Autodesk Inventor part; units mm, degrees
(part 3 of 6)
  line L1739 (82.2883, 113.1969) -> (82.3936, 113.3698)
  line L1740 (82.3936, 113.3698) -> (82.5145, 113.5317)
  line L1741 (82.5145, 113.5317) -> (82.6499, 113.6806)
  line L1742 (82.6499, 113.6806) -> (82.7991, 113.8163)
  line L1743 (82.7991, 113.8163) -> (82.9608, 113.9372)
  line L1744 (82.9608, 113.9372) -> (83.1339, 114.0423)
  line L1745 (83.1339, 114.0423) -> (83.3176, 114.1308)
  line L1746 (83.3176, 114.1308) -> (83.5105, 114.2015)
  line L1747 (83.5105, 114.2015) -> (83.7117, 114.2531)
  line L1748 (83.7117, 114.2531) -> (83.9201, 114.2848)
  line L1749 (83.9201, 114.2848) -> (84.1349, 114.2959)
  line L1750 (84.1349, 114.2959) -> (84.3495, 114.2848)
  line L1751 (84.3495, 114.2848) -> (84.5581, 114.2531)
  line L1752 (84.5581, 114.2531) -> (84.7593, 114.2015)
  line L1753 (84.7593, 114.2015) -> (84.9523, 114.1308)
  line L1754 (84.9523, 114.1308) -> (85.1359, 114.0423)
  line L1755 (85.1359, 114.0423) -> (85.309, 113.9372)
  line L1756 (85.309, 113.9372) -> (85.4708, 113.8163)
  line L1757 (85.4708, 113.8163) -> (85.6198, 113.6806)
  line L1758 (85.6198, 113.6806) -> (85.7553, 113.5317)
  line L1759 (85.7553, 113.5317) -> (85.8762, 113.3698)
  line L1760 (85.8762, 113.3698) -> (85.9815, 113.1969)
  line L1761 (85.9815, 113.1969) -> (86.0699, 113.0133)
  line L1762 (86.0699, 113.0133) -> (86.1405, 112.8203)
  line L1763 (86.1405, 112.8203) -> (86.1922, 112.6191)
  line L1764 (86.1922, 112.6191) -> (86.224, 112.4104)
  line L1765 (86.224, 112.4104) -> (86.2349, 112.1957)
  line L1766 (86.2349, 112.1957) -> (86.224, 111.9811)
  line L1767 (86.224, 111.9811) -> (86.1922, 111.7727)
  line L1768 (86.1922, 111.7727) -> (86.1405, 111.5711)
  line L1769 (86.1405, 111.5711) -> (86.0699, 111.3782)
  line L1770 (86.0699, 111.3782) -> (85.9815, 111.1949)
  line L1771 (85.9815, 111.1949) -> (85.8762, 111.0216)
  line L1772 (85.8762, 111.0216) -> (85.7553, 110.8601)
  line L1773 (85.7553, 110.8601) -> (85.6198, 110.7109)
  line L1774 (85.6198, 110.7109) -> (85.4708, 110.5752)
  line L1775 (85.4708, 110.5752) -> (85.309, 110.4546)
  line L1776 (85.309, 110.4546) -> (85.1359, 110.3492)
  line L1777 (85.1359, 110.3492) -> (84.9523, 110.261)
  line L1778 (84.9523, 110.261) -> (84.7593, 110.1903)
  line L1779 (84.7593, 110.1903) -> (84.5581, 110.1383)
  line L1780 (84.5581, 110.1383) -> (84.3495, 110.1066)
  line L1781 (84.3495, 110.1066) -> (84.1349, 110.0956)
  line L1782 (84.1349, 110.0956) -> (83.9201, 110.1066)
  line L1783 (83.9201, 110.1066) -> (83.7117, 110.1383)
  line L1784 (83.7117, 110.1383) -> (83.5105, 110.1903)
  line L1785 (83.5105, 110.1903) -> (83.3176, 110.261)
  line L1786 (83.3176, 110.261) -> (83.1339, 110.3492)
  line L1787 (83.1339, 110.3492) -> (82.9608, 110.4546)
  line L1788 (82.9608, 110.4546) -> (82.7991, 110.5752)
  line L1789 (82.7991, 110.5752) -> (82.6499, 110.7109)
  line L1790 (82.6499, 110.7109) -> (82.5145, 110.8601)
  line L1791 (82.5145, 110.8601) -> (82.3936, 111.0216)
  line L1792 (82.3936, 111.0216) -> (82.2883, 111.1949)
  line L1793 (82.2883, 111.1949) -> (82.2, 111.3782)
  line L1794 (82.2, 111.3782) -> (82.1294, 111.5711)
  line L1795 (82.1294, 111.5711) -> (82.0775, 111.7727)
  line L1796 (82.0775, 111.7727) -> (82.0458, 111.9811)
  line L1797 (82.0458, 111.9811) -> (82.035, 112.1957)
  line L1798 (12.0344, 112.1957) -> (12.0453, 112.4104)
  line L1799 (12.0453, 112.4104) -> (12.0771, 112.6191)
  line L1800 (12.0771, 112.6191) -> (12.1288, 112.8203)
  line L1801 (12.1288, 112.8203) -> (12.1994, 113.0133)
  line L1802 (12.1994, 113.0133) -> (12.288, 113.1969)
  line L1803 (12.288, 113.1969) -> (12.393, 113.3698)
  line L1804 (12.393, 113.3698) -> (12.514, 113.5317)
  line L1805 (12.514, 113.5317) -> (12.6495, 113.6806)
  line L1806 (12.6495, 113.6806) -> (12.7987, 113.8163)
  line L1807 (12.7987, 113.8163) -> (12.9603, 113.9372)
  line L1808 (12.9603, 113.9372) -> (13.1334, 114.0423)
  line L1809 (13.1334, 114.0423) -> (13.317, 114.1308)
  line L1810 (13.317, 114.1308) -> (13.5099, 114.2015)
  line L1811 (13.5099, 114.2015) -> (13.7111, 114.2531)
  line L1812 (13.7111, 114.2531) -> (13.9197, 114.2848)
  line L1813 (13.9197, 114.2848) -> (14.1344, 114.2959)
  line L1814 (14.1344, 114.2959) -> (14.3492, 114.2848)
  line L1815 (14.3492, 114.2848) -> (14.5576, 114.2531)
  line L1816 (14.5576, 114.2531) -> (14.759, 114.2015)
  line L1817 (14.759, 114.2015) -> (14.9519, 114.1308)
  line L1818 (14.9519, 114.1308) -> (15.1355, 114.0423)
  line L1819 (15.1355, 114.0423) -> (15.3086, 113.9372)
  line L1820 (15.3086, 113.9372) -> (15.4702, 113.8163)
  line L1821 (15.4702, 113.8163) -> (15.6194, 113.6806)
  line L1822 (15.6194, 113.6806) -> (15.7549, 113.5317)
  line L1823 (15.7549, 113.5317) -> (15.8759, 113.3698)
  line L1824 (15.8759, 113.3698) -> (15.9809, 113.1969)
  line L1825 (15.9809, 113.1969) -> (16.0695, 113.0133)
  line L1826 (16.0695, 113.0133) -> (16.1401, 112.8203)
  line L1827 (16.1401, 112.8203) -> (16.1918, 112.6191)
  line L1828 (16.1918, 112.6191) -> (16.2236, 112.4104)
  line L1829 (16.2236, 112.4104) -> (16.2345, 112.1957)
  line L1830 (16.2345, 112.1957) -> (16.2236, 111.9811)
  line L1831 (16.2236, 111.9811) -> (16.1918, 111.7727)
  line L1832 (16.1918, 111.7727) -> (16.1401, 111.5711)
  line L1833 (16.1401, 111.5711) -> (16.0695, 111.3782)
  line L1834 (16.0695, 111.3782) -> (15.9809, 111.1949)
  line L1835 (15.9809, 111.1949) -> (15.8759, 111.0216)
  line L1836 (15.8759, 111.0216) -> (15.7549, 110.8601)
  line L1837 (15.7549, 110.8601) -> (15.6194, 110.7109)
  line L1838 (15.6194, 110.7109) -> (15.4702, 110.5752)
  line L1839 (15.4702, 110.5752) -> (15.3086, 110.4546)
  line L1840 (15.3086, 110.4546) -> (15.1355, 110.3492)
  line L1841 (15.1355, 110.3492) -> (14.9519, 110.261)
  line L1842 (14.9519, 110.261) -> (14.759, 110.1903)
  line L1843 (14.759, 110.1903) -> (14.5576, 110.1383)
  line L1844 (14.5576, 110.1383) -> (14.3492, 110.1066)
  line L1845 (14.3492, 110.1066) -> (14.1344, 110.0956)
  line L1846 (14.1344, 110.0956) -> (13.9197, 110.1066)
  line L1847 (13.9197, 110.1066) -> (13.7111, 110.1383)
  line L1848 (13.7111, 110.1383) -> (13.5099, 110.1903)
  line L1849 (13.5099, 110.1903) -> (13.317, 110.261)
  line L1850 (13.317, 110.261) -> (13.1334, 110.3492)
  line L1851 (13.1334, 110.3492) -> (12.9603, 110.4546)
  line L1852 (12.9603, 110.4546) -> (12.7987, 110.5752)
  line L1853 (12.7987, 110.5752) -> (12.6495, 110.7109)
  line L1854 (12.6495, 110.7109) -> (12.514, 110.8601)
  line L1855 (12.514, 110.8601) -> (12.393, 111.0216)
  line L1856 (12.393, 111.0216) -> (12.288, 111.1949)
  line L1857 (12.288, 111.1949) -> (12.1994, 111.3782)
  line L1858 (12.1994, 111.3782) -> (12.1288, 111.5711)
  line L1859 (12.1288, 111.5711) -> (12.0771, 111.7727)
  line L1860 (12.0771, 111.7727) -> (12.0453, 111.9811)
  line L1861 (12.0453, 111.9811) -> (12.0344, 112.1957)
  line L1862 (26.0365, 112.1957) -> (26.0473, 112.4104)
  line L1863 (26.0473, 112.4104) -> (26.0792, 112.6191)
  line L1864 (26.0792, 112.6191) -> (26.1309, 112.8203)
  line L1865 (26.1309, 112.8203) -> (26.2015, 113.0133)
  line L1866 (26.2015, 113.0133) -> (26.2899, 113.1969)
  line L1867 (26.2899, 113.1969) -> (26.3951, 113.3698)
  line L1868 (26.3951, 113.3698) -> (26.516, 113.5317)
  line L1869 (26.516, 113.5317) -> (26.6516, 113.6806)
  line L1870 (26.6516, 113.6806) -> (26.8006, 113.8163)
  line L1871 (26.8006, 113.8163) -> (26.9624, 113.9372)
  line L1872 (26.9624, 113.9372) -> (27.1355, 114.0423)
  line L1873 (27.1355, 114.0423) -> (27.3191, 114.1308)
  line L1874 (27.3191, 114.1308) -> (27.512, 114.2015)
  line L1875 (27.512, 114.2015) -> (27.7132, 114.2531)
  line L1876 (27.7132, 114.2531) -> (27.9218, 114.2848)
  line L1877 (27.9218, 114.2848) -> (28.1364, 114.2959)
  line L1878 (28.1364, 114.2959) -> (28.3512, 114.2848)
  line L1879 (28.3512, 114.2848) -> (28.5597, 114.2531)
  line L1880 (28.5597, 114.2531) -> (28.7609, 114.2015)
  line L1881 (28.7609, 114.2015) -> (28.954, 114.1308)
  line L1882 (28.954, 114.1308) -> (29.1374, 114.0423)
  line L1883 (29.1374, 114.0423) -> (29.3105, 113.9372)
  line L1884 (29.3105, 113.9372) -> (29.4723, 113.8163)
  line L1885 (29.4723, 113.8163) -> (29.6214, 113.6806)
  line L1886 (29.6214, 113.6806) -> (29.7568, 113.5317)
  line L1887 (29.7568, 113.5317) -> (29.8778, 113.3698)
  line L1888 (29.8778, 113.3698) -> (29.983, 113.1969)
  line L1889 (29.983, 113.1969) -> (30.0714, 113.0133)
  line L1890 (30.0714, 113.0133) -> (30.142, 112.8203)
  line L1891 (30.142, 112.8203) -> (30.1939, 112.6191)
  line L1892 (30.1939, 112.6191) -> (30.2255, 112.4104)
  line L1893 (30.2255, 112.4104) -> (30.2364, 112.1957)
  line L1894 (30.2364, 112.1957) -> (30.2255, 111.9811)
  line L1895 (30.2255, 111.9811) -> (30.1939, 111.7727)
  line L1896 (30.1939, 111.7727) -> (30.142, 111.5711)
  line L1897 (30.142, 111.5711) -> (30.0714, 111.3782)
  line L1898 (30.0714, 111.3782) -> (29.983, 111.1949)
  line L1899 (29.983, 111.1949) -> (29.8778, 111.0216)
  line L1900 (29.8778, 111.0216) -> (29.7568, 110.8601)
  line L1901 (29.7568, 110.8601) -> (29.6214, 110.7109)
  line L1902 (29.6214, 110.7109) -> (29.4723, 110.5752)
  line L1903 (29.4723, 110.5752) -> (29.3105, 110.4546)
  line L1904 (29.3105, 110.4546) -> (29.1374, 110.3492)
  line L1905 (29.1374, 110.3492) -> (28.954, 110.261)
  line L1906 (28.954, 110.261) -> (28.7609, 110.1903)
  line L1907 (28.7609, 110.1903) -> (28.5597, 110.1383)
  line L1908 (28.5597, 110.1383) -> (28.3512, 110.1066)
  line L1909 (28.3512, 110.1066) -> (28.1364, 110.0956)
  line L1910 (28.1364, 110.0956) -> (27.9218, 110.1066)
  line L1911 (27.9218, 110.1066) -> (27.7132, 110.1383)
  line L1912 (27.7132, 110.1383) -> (27.512, 110.1903)
  line L1913 (27.512, 110.1903) -> (27.3191, 110.261)
  line L1914 (27.3191, 110.261) -> (27.1355, 110.3492)
  line L1915 (27.1355, 110.3492) -> (26.9624, 110.4546)
  line L1916 (26.9624, 110.4546) -> (26.8006, 110.5752)
  line L1917 (26.8006, 110.5752) -> (26.6516, 110.7109)
  line L1918 (26.6516, 110.7109) -> (26.516, 110.8601)
  line L1919 (26.516, 110.8601) -> (26.3951, 111.0216)
  line L1920 (26.3951, 111.0216) -> (26.2899, 111.1949)
  line L1921 (26.2899, 111.1949) -> (26.2015, 111.3782)
  line L1922 (26.2015, 111.3782) -> (26.1309, 111.5711)
  line L1923 (26.1309, 111.5711) -> (26.0792, 111.7727)
  line L1924 (26.0792, 111.7727) -> (26.0473, 111.9811)
  line L1925 (26.0473, 111.9811) -> (26.0365, 112.1957)
  line L1926 (40.0355, 112.1957) -> (40.0463, 112.4104)
  line L1927 (40.0463, 112.4104) -> (40.0782, 112.6191)
  line L1928 (40.0782, 112.6191) -> (40.1299, 112.8203)
  line L1929 (40.1299, 112.8203) -> (40.2005, 113.0133)
  line L1930 (40.2005, 113.0133) -> (40.289, 113.1969)
  line L1931 (40.289, 113.1969) -> (40.3941, 113.3698)
  line L1932 (40.3941, 113.3698) -> (40.515, 113.5317)
  line L1933 (40.515, 113.5317) -> (40.6506, 113.6806)
  line L1934 (40.6506, 113.6806) -> (40.7997, 113.8163)
  line L1935 (40.7997, 113.8163) -> (40.9613, 113.9372)
  line L1936 (40.9613, 113.9372) -> (41.1344, 114.0423)
  line L1937 (41.1344, 114.0423) -> (41.3181, 114.1308)
  line L1938 (41.3181, 114.1308) -> (41.511, 114.2015)
  line L1939 (41.511, 114.2015) -> (41.7122, 114.2531)
  line L1940 (41.7122, 114.2531) -> (41.9208, 114.2848)
  line L1941 (41.9208, 114.2848) -> (42.1354, 114.2959)
  line L1942 (42.1354, 114.2959) -> (42.3502, 114.2848)
  line L1943 (42.3502, 114.2848) -> (42.5586, 114.2531)
  line L1944 (42.5586, 114.2531) -> (42.76, 114.2015)
  line L1945 (42.76, 114.2015) -> (42.9529, 114.1308)
  line L1946 (42.9529, 114.1308) -> (43.1364, 114.0423)
  line L1947 (43.1364, 114.0423) -> (43.3097, 113.9372)
  line L1948 (43.3097, 113.9372) -> (43.4712, 113.8163)
  line L1949 (43.4712, 113.8163) -> (43.6204, 113.6806)
  line L1950 (43.6204, 113.6806) -> (43.756, 113.5317)
  line L1951 (43.756, 113.5317) -> (43.8769, 113.3698)
  line L1952 (43.8769, 113.3698) -> (43.982, 113.1969)
  line L1953 (43.982, 113.1969) -> (44.0705, 113.0133)
  line L1954 (44.0705, 113.0133) -> (44.1411, 112.8203)
  line L1955 (44.1411, 112.8203) -> (44.1928, 112.6191)
  line L1956 (44.1928, 112.6191) -> (44.2247, 112.4104)
  line L1957 (44.2247, 112.4104) -> (44.2355, 112.1957)
  line L1958 (44.2355, 112.1957) -> (44.2247, 111.9811)
  line L1959 (44.2247, 111.9811) -> (44.1928, 111.7727)
  line L1960 (44.1928, 111.7727) -> (44.1411, 111.5711)
  line L1961 (44.1411, 111.5711) -> (44.0705, 111.3782)
  line L1962 (44.0705, 111.3782) -> (43.982, 111.1949)
  line L1963 (43.982, 111.1949) -> (43.8769, 111.0216)
  line L1964 (43.8769, 111.0216) -> (43.756, 110.8601)
  line L1965 (43.756, 110.8601) -> (43.6204, 110.7109)
  line L1966 (43.6204, 110.7109) -> (43.4712, 110.5752)
  line L1967 (43.4712, 110.5752) -> (43.3097, 110.4546)
  line L1968 (43.3097, 110.4546) -> (43.1364, 110.3492)
  line L1969 (43.1364, 110.3492) -> (42.9529, 110.261)
  line L1970 (42.9529, 110.261) -> (42.76, 110.1903)
  line L1971 (42.76, 110.1903) -> (42.5586, 110.1383)
  line L1972 (42.5586, 110.1383) -> (42.3502, 110.1066)
  line L1973 (42.3502, 110.1066) -> (42.1354, 110.0956)
  line L1974 (42.1354, 110.0956) -> (41.9208, 110.1066)
  line L1975 (41.9208, 110.1066) -> (41.7122, 110.1383)
  line L1976 (41.7122, 110.1383) -> (41.511, 110.1903)
  line L1977 (41.511, 110.1903) -> (41.3181, 110.261)
  line L1978 (41.3181, 110.261) -> (41.1344, 110.3492)
  line L1979 (41.1344, 110.3492) -> (40.9613, 110.4546)
  line L1980 (40.9613, 110.4546) -> (40.7997, 110.5752)
  line L1981 (40.7997, 110.5752) -> (40.6506, 110.7109)
  line L1982 (40.6506, 110.7109) -> (40.515, 110.8601)
  line L1983 (40.515, 110.8601) -> (40.3941, 111.0216)
  line L1984 (40.3941, 111.0216) -> (40.289, 111.1949)
  line L1985 (40.289, 111.1949) -> (40.2005, 111.3782)
  line L1986 (40.2005, 111.3782) -> (40.1299, 111.5711)
  line L1987 (40.1299, 111.5711) -> (40.0782, 111.7727)
  line L1988 (40.0782, 111.7727) -> (40.0463, 111.9811)
  line L1989 (40.0463, 111.9811) -> (40.0355, 112.1957)
  line L1990 (54.0346, 112.1957) -> (54.0455, 112.4104)
  line L1991 (54.0455, 112.4104) -> (54.0773, 112.6191)
  line L1992 (54.0773, 112.6191) -> (54.1292, 112.8203)
  line L1993 (54.1292, 112.8203) -> (54.1996, 113.0133)
  line L1994 (54.1996, 113.0133) -> (54.2882, 113.1969)
  line L1995 (54.2882, 113.1969) -> (54.3934, 113.3698)
  line L1996 (54.3934, 113.3698) -> (54.5142, 113.5317)
  line L1997 (54.5142, 113.5317) -> (54.6497, 113.6806)
  line L1998 (54.6497, 113.6806) -> (54.7989, 113.8163)
  line L1999 (54.7989, 113.8163) -> (54.9605, 113.9372)
  line L2000 (54.9605, 113.9372) -> (55.1338, 114.0423)
  line L2001 (55.1338, 114.0423) -> (55.3172, 114.1308)
  line L2002 (55.3172, 114.1308) -> (55.5101, 114.2015)
  line L2003 (55.5101, 114.2015) -> (55.7115, 114.2531)
  line L2004 (55.7115, 114.2531) -> (55.9199, 114.2848)
  line L2005 (55.9199, 114.2848) -> (56.1347, 114.2959)
  line L2006 (56.1347, 114.2959) -> (56.3494, 114.2848)
  line L2007 (56.3494, 114.2848) -> (56.558, 114.2531)
  line L2008 (56.558, 114.2531) -> (56.7592, 114.2015)
  line L2009 (56.7592, 114.2015) -> (56.9521, 114.1308)
  line L2010 (56.9521, 114.1308) -> (57.1357, 114.0423)
  line L2011 (57.1357, 114.0423) -> (57.3088, 113.9372)
  line L2012 (57.3088, 113.9372) -> (57.4704, 113.8163)
  line L2013 (57.4704, 113.8163) -> (57.6196, 113.6806)
  line L2014 (57.6196, 113.6806) -> (57.7551, 113.5317)
  line L2015 (57.7551, 113.5317) -> (57.8761, 113.3698)
  line L2016 (57.8761, 113.3698) -> (57.9813, 113.1969)
  line L2017 (57.9813, 113.1969) -> (58.0697, 113.0133)
  line L2018 (58.0697, 113.0133) -> (58.1403, 112.8203)
  line L2019 (58.1403, 112.8203) -> (58.192, 112.6191)
  line L2020 (58.192, 112.6191) -> (58.2238, 112.4104)
  line L2021 (58.2238, 112.4104) -> (58.2347, 112.1957)
  line L2022 (58.2347, 112.1957) -> (58.2238, 111.9811)
  line L2023 (58.2238, 111.9811) -> (58.192, 111.7727)
  line L2024 (58.192, 111.7727) -> (58.1403, 111.5711)
  line L2025 (58.1403, 111.5711) -> (58.0697, 111.3782)
  line L2026 (58.0697, 111.3782) -> (57.9813, 111.1949)
  line L2027 (57.9813, 111.1949) -> (57.8761, 111.0216)
  line L2028 (57.8761, 111.0216) -> (57.7551, 110.8601)
  line L2029 (57.7551, 110.8601) -> (57.6196, 110.7109)
  line L2030 (57.6196, 110.7109) -> (57.4704, 110.5752)
  line L2031 (57.4704, 110.5752) -> (57.3088, 110.4546)
  line L2032 (57.3088, 110.4546) -> (57.1357, 110.3492)
  line L2033 (57.1357, 110.3492) -> (56.9521, 110.261)
  line L2034 (56.9521, 110.261) -> (56.7592, 110.1903)
  line L2035 (56.7592, 110.1903) -> (56.558, 110.1383)
  line L2036 (56.558, 110.1383) -> (56.3494, 110.1066)
  line L2037 (56.3494, 110.1066) -> (56.1347, 110.0956)
  line L2038 (56.1347, 110.0956) -> (55.9199, 110.1066)
  line L2039 (55.9199, 110.1066) -> (55.7115, 110.1383)
  line L2040 (55.7115, 110.1383) -> (55.5101, 110.1903)
  line L2041 (55.5101, 110.1903) -> (55.3172, 110.261)
  line L2042 (55.3172, 110.261) -> (55.1338, 110.3492)
  line L2043 (55.1338, 110.3492) -> (54.9605, 110.4546)
  line L2044 (54.9605, 110.4546) -> (54.7989, 110.5752)
  line L2045 (54.7989, 110.5752) -> (54.6497, 110.7109)
  line L2046 (54.6497, 110.7109) -> (54.5142, 110.8601)
  line L2047 (54.5142, 110.8601) -> (54.3934, 111.0216)
  line L2048 (54.3934, 111.0216) -> (54.2882, 111.1949)
  line L2049 (54.2882, 111.1949) -> (54.1996, 111.3782)
  line L2050 (54.1996, 111.3782) -> (54.1292, 111.5711)
  line L2051 (54.1292, 111.5711) -> (54.0773, 111.7727)
  line L2052 (54.0773, 111.7727) -> (54.0455, 111.9811)
  line L2053 (54.0455, 111.9811) -> (54.0346, 112.1957)
  line L2054 (96.0253, 112.1957) -> (96.0362, 112.4104)
  line L2055 (96.0362, 112.4104) -> (96.0679, 112.6191)
  line L2056 (96.0679, 112.6191) -> (96.1197, 112.8203)
  line L2057 (96.1197, 112.8203) -> (96.1903, 113.0133)
  line L2058 (96.1903, 113.0133) -> (96.2787, 113.1969)
  line L2059 (96.2787, 113.1969) -> (96.384, 113.3698)
  line L2060 (96.384, 113.3698) -> (96.5049, 113.5317)
  line L2061 (96.5049, 113.5317) -> (96.6403, 113.6806)
  line L2062 (96.6403, 113.6806) -> (96.7894, 113.8163)
  line L2063 (96.7894, 113.8163) -> (96.9512, 113.9372)
  line L2064 (96.9512, 113.9372) -> (97.1243, 114.0423)
  line L2065 (97.1243, 114.0423) -> (97.3079, 114.1308)
  line L2066 (97.3079, 114.1308) -> (97.5009, 114.2015)
  line L2067 (97.5009, 114.2015) -> (97.702, 114.2531)
  line L2068 (97.702, 114.2531) -> (97.9105, 114.2848)
  line L2069 (97.9105, 114.2848) -> (98.1253, 114.2959)
  line L2070 (98.1253, 114.2959) -> (98.3399, 114.2848)
  line L2071 (98.3399, 114.2848) -> (98.5485, 114.2531)
  line L2072 (98.5485, 114.2531) -> (98.7497, 114.2015)
  line L2073 (98.7497, 114.2015) -> (98.9426, 114.1308)
  line L2074 (98.9426, 114.1308) -> (99.1262, 114.0423)
  line L2075 (99.1262, 114.0423) -> (99.2994, 113.9372)
  line L2076 (99.2994, 113.9372) -> (99.4611, 113.8163)
  line L2077 (99.4611, 113.8163) -> (99.6101, 113.6806)
  line L2078 (99.6101, 113.6806) -> (99.7457, 113.5317)
  line L2079 (99.7457, 113.5317) -> (99.8666, 113.3698)
  line L2080 (99.8666, 113.3698) -> (99.9718, 113.1969)
  line L2081 (99.9718, 113.1969) -> (100.0602, 113.0133)
  line L2082 (100.0602, 113.0133) -> (100.1308, 112.8203)
  line L2083 (100.1308, 112.8203) -> (100.1827, 112.6191)
  line L2084 (100.1827, 112.6191) -> (100.2144, 112.4104)
  line L2085 (100.2144, 112.4104) -> (100.2252, 112.1957)
  line L2086 (100.2252, 112.1957) -> (100.2144, 111.9811)
  line L2087 (100.2144, 111.9811) -> (100.1827, 111.7727)
  line L2088 (100.1827, 111.7727) -> (100.1308, 111.5711)
  line L2089 (100.1308, 111.5711) -> (100.0602, 111.3782)
  line L2090 (100.0602, 111.3782) -> (99.9718, 111.1949)
  line L2091 (99.9718, 111.1949) -> (99.8666, 111.0216)
  line L2092 (99.8666, 111.0216) -> (99.7457, 110.8601)
  line L2093 (99.7457, 110.8601) -> (99.6101, 110.7109)
  line L2094 (99.6101, 110.7109) -> (99.4611, 110.5752)
  line L2095 (99.4611, 110.5752) -> (99.2994, 110.4546)
  line L2096 (99.2994, 110.4546) -> (99.1262, 110.3492)
  line L2097 (99.1262, 110.3492) -> (98.9426, 110.261)
  line L2098 (98.9426, 110.261) -> (98.7497, 110.1903)
  line L2099 (98.7497, 110.1903) -> (98.5485, 110.1383)
  line L2100 (98.5485, 110.1383) -> (98.3399, 110.1066)
  line L2101 (98.3399, 110.1066) -> (98.1253, 110.0956)
  line L2102 (98.1253, 110.0956) -> (97.9105, 110.1066)
  line L2103 (97.9105, 110.1066) -> (97.702, 110.1383)
  line L2104 (97.702, 110.1383) -> (97.5009, 110.1903)
  line L2105 (97.5009, 110.1903) -> (97.3079, 110.261)
  line L2106 (97.3079, 110.261) -> (97.1243, 110.3492)
  line L2107 (97.1243, 110.3492) -> (96.9512, 110.4546)
  line L2108 (96.9512, 110.4546) -> (96.7894, 110.5752)
  line L2109 (96.7894, 110.5752) -> (96.6403, 110.7109)
  line L2110 (96.6403, 110.7109) -> (96.5049, 110.8601)
  line L2111 (96.5049, 110.8601) -> (96.384, 111.0216)
  line L2112 (96.384, 111.0216) -> (96.2787, 111.1949)
  line L2113 (96.2787, 111.1949) -> (96.1903, 111.3782)
  line L2114 (96.1903, 111.3782) -> (96.1197, 111.5711)
  line L2115 (96.1197, 111.5711) -> (96.0679, 111.7727)
  line L2116 (96.0679, 111.7727) -> (96.0362, 111.9811)
  line L2117 (96.0362, 111.9811) -> (96.0253, 112.1957)
  line L2118 (110.0253, 112.1957) -> (110.0363, 112.4104)
  line L2119 (110.0363, 112.4104) -> (110.068, 112.6191)
  line L2120 (110.068, 112.6191) -> (110.1197, 112.8203)
  line L2121 (110.1197, 112.8203) -> (110.1903, 113.0133)
  line L2122 (110.1903, 113.0133) -> (110.2789, 113.1969)
  line L2123 (110.2789, 113.1969) -> (110.384, 113.3698)
  line L2124 (110.384, 113.3698) -> (110.5049, 113.5317)
  line L2125 (110.5049, 113.5317) -> (110.6406, 113.6806)
  line L2126 (110.6406, 113.6806) -> (110.7898, 113.8163)
  line L2127 (110.7898, 113.8163) -> (110.9514, 113.9372)
  line L2128 (110.9514, 113.9372) -> (111.1243, 114.0423)
  line L2129 (111.1243, 114.0423) -> (111.3079, 114.1308)
  line L2130 (111.3079, 114.1308) -> (111.5009, 114.2015)
  line L2131 (111.5009, 114.2015) -> (111.7024, 114.2531)
  line L2132 (111.7024, 114.2531) -> (111.9108, 114.2848)
  line L2133 (111.9108, 114.2848) -> (112.1255, 114.2959)
  line L2134 (112.1255, 114.2959) -> (112.3401, 114.2848)
  line L2135 (112.3401, 114.2848) -> (112.5489, 114.2531)
  line L2136 (112.5489, 114.2531) -> (112.7501, 114.2015)
  line L2137 (112.7501, 114.2015) -> (112.943, 114.1308)
  line L2138 (112.943, 114.1308) -> (113.1266, 114.0423)
  line L2139 (113.1266, 114.0423) -> (113.2995, 113.9372)
  line L2140 (113.2995, 113.9372) -> (113.4611, 113.8163)
  line L2141 (113.4611, 113.8163) -> (113.6103, 113.6806)
  line L2142 (113.6103, 113.6806) -> (113.746, 113.5317)
  line L2143 (113.746, 113.5317) -> (113.867, 113.3698)
  line L2144 (113.867, 113.3698) -> (113.972, 113.1969)
  line L2145 (113.972, 113.1969) -> (114.0606, 113.0133)
  line L2146 (114.0606, 113.0133) -> (114.1312, 112.8203)
  line L2147 (114.1312, 112.8203) -> (114.1829, 112.6191)
  line L2148 (114.1829, 112.6191) -> (114.2146, 112.4104)
  line L2149 (114.2146, 112.4104) -> (114.2256, 112.1957)
  line L2150 (114.2256, 112.1957) -> (114.2146, 111.9811)
  line L2151 (114.2146, 111.9811) -> (114.1829, 111.7727)
  line L2152 (114.1829, 111.7727) -> (114.1312, 111.5711)
  line L2153 (114.1312, 111.5711) -> (114.0606, 111.3782)
  line L2154 (114.0606, 111.3782) -> (113.972, 111.1949)
  line L2155 (113.972, 111.1949) -> (113.867, 111.0216)
  line L2156 (113.867, 111.0216) -> (113.746, 110.8601)
  line L2157 (113.746, 110.8601) -> (113.6103, 110.7109)
  line L2158 (113.6103, 110.7109) -> (113.4611, 110.5752)
  line L2159 (113.4611, 110.5752) -> (113.2995, 110.4546)
  line L2160 (113.2995, 110.4546) -> (113.1266, 110.3492)
  line L2161 (113.1266, 110.3492) -> (112.943, 110.261)
  line L2162 (112.943, 110.261) -> (112.7501, 110.1903)
  line L2163 (112.7501, 110.1903) -> (112.5489, 110.1383)
  line L2164 (112.5489, 110.1383) -> (112.3401, 110.1066)
  line L2165 (112.3401, 110.1066) -> (112.1255, 110.0956)
  line L2166 (112.1255, 110.0956) -> (111.9108, 110.1066)
  line L2167 (111.9108, 110.1066) -> (111.7024, 110.1383)
  line L2168 (111.7024, 110.1383) -> (111.5009, 110.1903)
  line L2169 (111.5009, 110.1903) -> (111.3079, 110.261)
  line L2170 (111.3079, 110.261) -> (111.1243, 110.3492)
  line L2171 (111.1243, 110.3492) -> (110.9514, 110.4546)
  line L2172 (110.9514, 110.4546) -> (110.7898, 110.5752)
  line L2173 (110.7898, 110.5752) -> (110.6406, 110.7109)
  line L2174 (110.6406, 110.7109) -> (110.5049, 110.8601)
  line L2175 (110.5049, 110.8601) -> (110.384, 111.0216)
  line L2176 (110.384, 111.0216) -> (110.2789, 111.1949)
  line L2177 (110.2789, 111.1949) -> (110.1903, 111.3782)
  line L2178 (110.1903, 111.3782) -> (110.1197, 111.5711)
  line L2179 (110.1197, 111.5711) -> (110.068, 111.7727)
  line L2180 (110.068, 111.7727) -> (110.0363, 111.9811)
  line L2181 (110.0363, 111.9811) -> (110.0253, 112.1957)
  line L2182 (54.0346, 185.1932) -> (54.0455, 185.408)
  line L2183 (54.0455, 185.408) -> (54.0773, 185.6164)
  line L2184 (54.0773, 185.6164) -> (54.1292, 185.8178)
  line L2185 (54.1292, 185.8178) -> (54.1996, 186.0107)
  line L2186 (54.1996, 186.0107) -> (54.2882, 186.1941)
  line L2187 (54.2882, 186.1941) -> (54.3934, 186.3673)
  line L2188 (54.3934, 186.3673) -> (54.5142, 186.529)
  line L2189 (54.5142, 186.529) -> (54.6497, 186.6782)
  line L2190 (54.6497, 186.6782) -> (54.7989, 186.8137)
  line L2191 (54.7989, 186.8137) -> (54.9605, 186.9345)
  line L2192 (54.9605, 186.9345) -> (55.1338, 187.0397)
  line L2193 (55.1338, 187.0397) -> (55.3172, 187.1281)
  line L2194 (55.3172, 187.1281) -> (55.5101, 187.1987)
  line L2195 (55.5101, 187.1987) -> (55.7115, 187.2506)
  line L2196 (55.7115, 187.2506) -> (55.9199, 187.2823)
  line L2197 (55.9199, 187.2823) -> (56.1347, 187.2931)
  line L2198 (56.1347, 187.2931) -> (56.3494, 187.2823)
  line L2199 (56.3494, 187.2823) -> (56.558, 187.2506)
  line L2200 (56.558, 187.2506) -> (56.7592, 187.1987)
  line L2201 (56.7592, 187.1987) -> (56.9521, 187.1281)
  line L2202 (56.9521, 187.1281) -> (57.1357, 187.0397)
  line L2203 (57.1357, 187.0397) -> (57.3088, 186.9345)
  line L2204 (57.3088, 186.9345) -> (57.4704, 186.8137)
  line L2205 (57.4704, 186.8137) -> (57.6196, 186.6782)
  line L2206 (57.6196, 186.6782) -> (57.7551, 186.529)
  line L2207 (57.7551, 186.529) -> (57.8761, 186.3673)
  line L2208 (57.8761, 186.3673) -> (57.9813, 186.1941)
  line L2209 (57.9813, 186.1941) -> (58.0697, 186.0107)
  line L2210 (58.0697, 186.0107) -> (58.1403, 185.8178)
  line L2211 (58.1403, 185.8178) -> (58.192, 185.6164)
  line L2212 (58.192, 185.6164) -> (58.2238, 185.408)
  line L2213 (58.2238, 185.408) -> (58.2347, 185.1932)
  line L2214 (58.2347, 185.1932) -> (58.2238, 184.9785)
  line L2215 (58.2238, 184.9785) -> (58.192, 184.7699)
  line L2216 (58.192, 184.7699) -> (58.1403, 184.5688)
  line L2217 (58.1403, 184.5688) -> (58.0697, 184.3758)
  line L2218 (58.0697, 184.3758) -> (57.9813, 184.1922)
  line L2219 (57.9813, 184.1922) -> (57.8761, 184.0191)
  line L2220 (57.8761, 184.0191) -> (57.7551, 183.8573)
  line L2221 (57.7551, 183.8573) -> (57.6196, 183.7083)
  line L2222 (57.6196, 183.7083) -> (57.4704, 183.5728)
  line L2223 (57.4704, 183.5728) -> (57.3088, 183.4519)
  line L2224 (57.3088, 183.4519) -> (57.1357, 183.3466)
  line L2225 (57.1357, 183.3466) -> (56.9521, 183.2582)
  line L2226 (56.9521, 183.2582) -> (56.7592, 183.1876)
  line L2227 (56.7592, 183.1876) -> (56.558, 183.1359)
  line L2228 (56.558, 183.1359) -> (56.3494, 183.1041)
  line L2229 (56.3494, 183.1041) -> (56.1347, 183.0932)
  line L2230 (56.1347, 183.0932) -> (55.9199, 183.1041)
  line L2231 (55.9199, 183.1041) -> (55.7115, 183.1359)
  line L2232 (55.7115, 183.1359) -> (55.5101, 183.1876)
  line L2233 (55.5101, 183.1876) -> (55.3172, 183.2582)
  line L2234 (55.3172, 183.2582) -> (55.1338, 183.3466)
  line L2235 (55.1338, 183.3466) -> (54.9605, 183.4519)
  line L2236 (54.9605, 183.4519) -> (54.7989, 183.5728)
  line L2237 (54.7989, 183.5728) -> (54.6497, 183.7083)
  line L2238 (54.6497, 183.7083) -> (54.5142, 183.8573)
  line L2239 (54.5142, 183.8573) -> (54.3934, 184.0191)
  line L2240 (54.3934, 184.0191) -> (54.2882, 184.1922)
  line L2241 (54.2882, 184.1922) -> (54.1996, 184.3758)
  line L2242 (54.1996, 184.3758) -> (54.1292, 184.5688)
  line L2243 (54.1292, 184.5688) -> (54.0773, 184.7699)
  line L2244 (54.0773, 184.7699) -> (54.0455, 184.9785)
  line L2245 (54.0455, 184.9785) -> (54.0346, 185.1932)
  line L2246 (82.035, 185.1932) -> (82.0458, 185.408)
  line L2247 (82.0458, 185.408) -> (82.0775, 185.6164)
  line L2248 (82.0775, 185.6164) -> (82.1294, 185.8178)
  line L2249 (82.1294, 185.8178) -> (82.2, 186.0107)
  line L2250 (82.2, 186.0107) -> (82.2883, 186.1941)
  line L2251 (82.2883, 186.1941) -> (82.3936, 186.3673)
  line L2252 (82.3936, 186.3673) -> (82.5145, 186.529)
  line L2253 (82.5145, 186.529) -> (82.6499, 186.6782)
  line L2254 (82.6499, 186.6782) -> (82.7991, 186.8137)
  line L2255 (82.7991, 186.8137) -> (82.9608, 186.9345)
  line L2256 (82.9608, 186.9345) -> (83.1339, 187.0397)
  line L2257 (83.1339, 187.0397) -> (83.3176, 187.1281)
  line L2258 (83.3176, 187.1281) -> (83.5105, 187.1987)
  line L2259 (83.5105, 187.1987) -> (83.7117, 187.2506)
  line L2260 (83.7117, 187.2506) -> (83.9201, 187.2823)
  line L2261 (83.9201, 187.2823) -> (84.1349, 187.2931)
  line L2262 (84.1349, 187.2931) -> (84.3495, 187.2823)
  line L2263 (84.3495, 187.2823) -> (84.5581, 187.2506)
  line L2264 (84.5581, 187.2506) -> (84.7593, 187.1987)
  line L2265 (84.7593, 187.1987) -> (84.9523, 187.1281)
  line L2266 (84.9523, 187.1281) -> (85.1359, 187.0397)
  line L2267 (85.1359, 187.0397) -> (85.309, 186.9345)
  line L2268 (85.309, 186.9345) -> (85.4708, 186.8137)
  line L2269 (85.4708, 186.8137) -> (85.6198, 186.6782)
  line L2270 (85.6198, 186.6782) -> (85.7553, 186.529)
  line L2271 (85.7553, 186.529) -> (85.8762, 186.3673)
  line L2272 (85.8762, 186.3673) -> (85.9815, 186.1941)
  line L2273 (85.9815, 186.1941) -> (86.0699, 186.0107)
  line L2274 (86.0699, 186.0107) -> (86.1405, 185.8178)
  line L2275 (86.1405, 185.8178) -> (86.1922, 185.6164)
  line L2276 (86.1922, 185.6164) -> (86.224, 185.408)
  line L2277 (86.224, 185.408) -> (86.2349, 185.1932)
  line L2278 (86.2349, 185.1932) -> (86.224, 184.9785)
  line L2279 (86.224, 184.9785) -> (86.1922, 184.7699)
  line L2280 (86.1922, 184.7699) -> (86.1405, 184.5688)
  line L2281 (86.1405, 184.5688) -> (86.0699, 184.3758)
  line L2282 (86.0699, 184.3758) -> (85.9815, 184.1922)
  line L2283 (85.9815, 184.1922) -> (85.8762, 184.0191)
  line L2284 (85.8762, 184.0191) -> (85.7553, 183.8573)
  line L2285 (85.7553, 183.8573) -> (85.6198, 183.7083)
  line L2286 (85.6198, 183.7083) -> (85.4708, 183.5728)
  line L2287 (85.4708, 183.5728) -> (85.309, 183.4519)
  line L2288 (85.309, 183.4519) -> (85.1359, 183.3466)
  line L2289 (85.1359, 183.3466) -> (84.9523, 183.2582)
  line L2290 (84.9523, 183.2582) -> (84.7593, 183.1876)
  line L2291 (84.7593, 183.1876) -> (84.5581, 183.1359)
  line L2292 (84.5581, 183.1359) -> (84.3495, 183.1041)
  line L2293 (84.3495, 183.1041) -> (84.1349, 183.0932)
  line L2294 (84.1349, 183.0932) -> (83.9201, 183.1041)
  line L2295 (83.9201, 183.1041) -> (83.7117, 183.1359)
  line L2296 (83.7117, 183.1359) -> (83.5105, 183.1876)
  line L2297 (83.5105, 183.1876) -> (83.3176, 183.2582)
  line L2298 (83.3176, 183.2582) -> (83.1339, 183.3466)
  line L2299 (83.1339, 183.3466) -> (82.9608, 183.4519)
  line L2300 (82.9608, 183.4519) -> (82.7991, 183.5728)
  line L2301 (82.7991, 183.5728) -> (82.6499, 183.7083)
  line L2302 (82.6499, 183.7083) -> (82.5145, 183.8573)
  line L2303 (82.5145, 183.8573) -> (82.3936, 184.0191)
  line L2304 (82.3936, 184.0191) -> (82.2883, 184.1922)
  line L2305 (82.2883, 184.1922) -> (82.2, 184.3758)
  line L2306 (82.2, 184.3758) -> (82.1294, 184.5688)
  line L2307 (82.1294, 184.5688) -> (82.0775, 184.7699)
  line L2308 (82.0775, 184.7699) -> (82.0458, 184.9785)
  line L2309 (82.0458, 184.9785) -> (82.035, 185.1932)
  line L2310 (68.0346, 185.1932) -> (68.0455, 185.408)
  line L2311 (68.0455, 185.408) -> (68.0772, 185.6164)
  line L2312 (68.0772, 185.6164) -> (68.129, 185.8178)
  line L2313 (68.129, 185.8178) -> (68.1996, 186.0107)
  line L2314 (68.1996, 186.0107) -> (68.288, 186.1941)
  line L2315 (68.288, 186.1941) -> (68.3932, 186.3673)
  line L2316 (68.3932, 186.3673) -> (68.5142, 186.529)
  line L2317 (68.5142, 186.529) -> (68.6496, 186.6782)
  line L2318 (68.6496, 186.6782) -> (68.7987, 186.8137)
  line L2319 (68.7987, 186.8137) -> (68.9605, 186.9345)
  line L2320 (68.9605, 186.9345) -> (69.1336, 187.0397)
  line L2321 (69.1336, 187.0397) -> (69.317, 187.1281)
  line L2322 (69.317, 187.1281) -> (69.5101, 187.1987)
  line L2323 (69.5101, 187.1987) -> (69.7113, 187.2506)
  line L2324 (69.7113, 187.2506) -> (69.9198, 187.2823)
  line L2325 (69.9198, 187.2823) -> (70.1346, 187.2931)
  line L2326 (70.1346, 187.2931) -> (70.3492, 187.2823)
  line L2327 (70.3492, 187.2823) -> (70.5578, 187.2506)
  line L2328 (70.5578, 187.2506) -> (70.759, 187.1987)
  line L2329 (70.759, 187.1987) -> (70.9519, 187.1281)
  line L2330 (70.9519, 187.1281) -> (71.1355, 187.0397)
  line L2331 (71.1355, 187.0397) -> (71.3087, 186.9345)
  line L2332 (71.3087, 186.9345) -> (71.4704, 186.8137)
  line L2333 (71.4704, 186.8137) -> (71.6194, 186.6782)
  line L2334 (71.6194, 186.6782) -> (71.755, 186.529)
  line L2335 (71.755, 186.529) -> (71.8759, 186.3673)
  line L2336 (71.8759, 186.3673) -> (71.9811, 186.1941)
  line L2337 (71.9811, 186.1941) -> (72.0695, 186.0107)
  line L2338 (72.0695, 186.0107) -> (72.1401, 185.8178)
  line L2339 (72.1401, 185.8178) -> (72.1918, 185.6164)
  line L2340 (72.1918, 185.6164) -> (72.2237, 185.408)
  line L2341 (72.2237, 185.408) -> (72.2345, 185.1932)
  line L2342 (72.2345, 185.1932) -> (72.2237, 184.9785)
  line L2343 (72.2237, 184.9785) -> (72.1918, 184.7699)
  line L2344 (72.1918, 184.7699) -> (72.1401, 184.5688)
  line L2345 (72.1401, 184.5688) -> (72.0695, 184.3758)
  line L2346 (72.0695, 184.3758) -> (71.9811, 184.1922)
  line L2347 (71.9811, 184.1922) -> (71.8759, 184.0191)
  line L2348 (71.8759, 184.0191) -> (71.755, 183.8573)
  line L2349 (71.755, 183.8573) -> (71.6194, 183.7083)
  line L2350 (71.6194, 183.7083) -> (71.4704, 183.5728)
  line L2351 (71.4704, 183.5728) -> (71.3087, 183.4519)
  line L2352 (71.3087, 183.4519) -> (71.1355, 183.3466)
  line L2353 (71.1355, 183.3466) -> (70.9519, 183.2582)
  line L2354 (70.9519, 183.2582) -> (70.759, 183.1876)
  line L2355 (70.759, 183.1876) -> (70.5578, 183.1359)
  line L2356 (70.5578, 183.1359) -> (70.3492, 183.1041)
  line L2357 (70.3492, 183.1041) -> (70.1346, 183.0932)
  line L2358 (70.1346, 183.0932) -> (69.9198, 183.1041)
  line L2359 (69.9198, 183.1041) -> (69.7113, 183.1359)
  line L2360 (69.7113, 183.1359) -> (69.5101, 183.1876)
  line L2361 (69.5101, 183.1876) -> (69.317, 183.2582)
  line L2362 (69.317, 183.2582) -> (69.1336, 183.3466)
  line L2363 (69.1336, 183.3466) -> (68.9605, 183.4519)
  line L2364 (68.9605, 183.4519) -> (68.7987, 183.5728)
  line L2365 (68.7987, 183.5728) -> (68.6496, 183.7083)
  line L2366 (68.6496, 183.7083) -> (68.5142, 183.8573)
  line L2367 (68.5142, 183.8573) -> (68.3932, 184.0191)
  line L2368 (68.3932, 184.0191) -> (68.288, 184.1922)
  line L2369 (68.288, 184.1922) -> (68.1996, 184.3758)
  line L2370 (68.1996, 184.3758) -> (68.129, 184.5688)
  line L2371 (68.129, 184.5688) -> (68.0772, 184.7699)
  line L2372 (68.0772, 184.7699) -> (68.0455, 184.9785)
  line L2373 (68.0455, 184.9785) -> (68.0346, 185.1932)
  line L2374 (96.0253, 185.1932) -> (96.0362, 185.408)
  line L2375 (96.0362, 185.408) -> (96.0679, 185.6164)
  line L2376 (96.0679, 185.6164) -> (96.1197, 185.8178)
  line L2377 (96.1197, 185.8178) -> (96.1903, 186.0107)
  line L2378 (96.1903, 186.0107) -> (96.2787, 186.1941)
  line L2379 (96.2787, 186.1941) -> (96.384, 186.3673)
  line L2380 (96.384, 186.3673) -> (96.5049, 186.529)
  line L2381 (96.5049, 186.529) -> (96.6403, 186.6782)
  line L2382 (96.6403, 186.6782) -> (96.7894, 186.8137)
  line L2383 (96.7894, 186.8137) -> (96.9512, 186.9345)
  line L2384 (96.9512, 186.9345) -> (97.1243, 187.0397)
  line L2385 (97.1243, 187.0397) -> (97.3079, 187.1281)
  line L2386 (97.3079, 187.1281) -> (97.5009, 187.1987)
  line L2387 (97.5009, 187.1987) -> (97.702, 187.2506)
  line L2388 (97.702, 187.2506) -> (97.9105, 187.2823)
  line L2389 (97.9105, 187.2823) -> (98.1253, 187.2931)
  line L2390 (98.1253, 187.2931) -> (98.3399, 187.2823)
  line L2391 (98.3399, 187.2823) -> (98.5485, 187.2506)
  line L2392 (98.5485, 187.2506) -> (98.7497, 187.1987)
  line L2393 (98.7497, 187.1987) -> (98.9426, 187.1281)
  line L2394 (98.9426, 187.1281) -> (99.1262, 187.0397)
  line L2395 (99.1262, 187.0397) -> (99.2994, 186.9345)
  line L2396 (99.2994, 186.9345) -> (99.4611, 186.8137)
  line L2397 (99.4611, 186.8137) -> (99.6101, 186.6782)
  line L2398 (99.6101, 186.6782) -> (99.7457, 186.529)
  line L2399 (99.7457, 186.529) -> (99.8666, 186.3673)
  line L2400 (99.8666, 186.3673) -> (99.9718, 186.1941)
  line L2401 (99.9718, 186.1941) -> (100.0602, 186.0107)
  line L2402 (100.0602, 186.0107) -> (100.1308, 185.8178)
  line L2403 (100.1308, 185.8178) -> (100.1827, 185.6164)
  line L2404 (100.1827, 185.6164) -> (100.2144, 185.408)
  line L2405 (100.2144, 185.408) -> (100.2252, 185.1932)
  line L2406 (100.2252, 185.1932) -> (100.2144, 184.9785)
  line L2407 (100.2144, 184.9785) -> (100.1827, 184.7699)
  line L2408 (100.1827, 184.7699) -> (100.1308, 184.5688)
  line L2409 (100.1308, 184.5688) -> (100.0602, 184.3758)
  line L2410 (100.0602, 184.3758) -> (99.9718, 184.1922)
  line L2411 (99.9718, 184.1922) -> (99.8666, 184.0191)
  line L2412 (99.8666, 184.0191) -> (99.7457, 183.8573)
  line L2413 (99.7457, 183.8573) -> (99.6101, 183.7083)
  line L2414 (99.6101, 183.7083) -> (99.4611, 183.5728)
  line L2415 (99.4611, 183.5728) -> (99.2994, 183.4519)
  line L2416 (99.2994, 183.4519) -> (99.1262, 183.3466)
  line L2417 (99.1262, 183.3466) -> (98.9426, 183.2582)
  line L2418 (98.9426, 183.2582) -> (98.7497, 183.1876)
  line L2419 (98.7497, 183.1876) -> (98.5485, 183.1359)
  line L2420 (98.5485, 183.1359) -> (98.3399, 183.1041)
  line L2421 (98.3399, 183.1041) -> (98.1253, 183.0932)
  line L2422 (98.1253, 183.0932) -> (97.9105, 183.1041)
  line L2423 (97.9105, 183.1041) -> (97.702, 183.1359)
  line L2424 (97.702, 183.1359) -> (97.5009, 183.1876)
  line L2425 (97.5009, 183.1876) -> (97.3079, 183.2582)
  line L2426 (97.3079, 183.2582) -> (97.1243, 183.3466)
  line L2427 (97.1243, 183.3466) -> (96.9512, 183.4519)
  line L2428 (96.9512, 183.4519) -> (96.7894, 183.5728)
  line L2429 (96.7894, 183.5728) -> (96.6403, 183.7083)
  line L2430 (96.6403, 183.7083) -> (96.5049, 183.8573)
  line L2431 (96.5049, 183.8573) -> (96.384, 184.0191)
  line L2432 (96.384, 184.0191) -> (96.2787, 184.1922)
  line L2433 (96.2787, 184.1922) -> (96.1903, 184.3758)
  line L2434 (96.1903, 184.3758) -> (96.1197, 184.5688)
  line L2435 (96.1197, 184.5688) -> (96.0679, 184.7699)
  line L2436 (96.0679, 184.7699) -> (96.0362, 184.9785)
  line L2437 (96.0362, 184.9785) -> (96.0253, 185.1932)
  line L2438 (110.0253, 185.1932) -> (110.0363, 185.408)
  line L2439 (110.0363, 185.408) -> (110.068, 185.6164)
  line L2440 (110.068, 185.6164) -> (110.1197, 185.8178)
  line L2441 (110.1197, 185.8178) -> (110.1903, 186.0107)
  line L2442 (110.1903, 186.0107) -> (110.2789, 186.1941)
  line L2443 (110.2789, 186.1941) -> (110.384, 186.3673)
  line L2444 (110.384, 186.3673) -> (110.5049, 186.529)
  line L2445 (110.5049, 186.529) -> (110.6406, 186.6782)
  line L2446 (110.6406, 186.6782) -> (110.7898, 186.8137)
  line L2447 (110.7898, 186.8137) -> (110.9514, 186.9345)
  line L2448 (110.9514, 186.9345) -> (111.1243, 187.0397)
  line L2449 (111.1243, 187.0397) -> (111.3079, 187.1281)
  line L2450 (111.3079, 187.1281) -> (111.5009, 187.1987)
  line L2451 (111.5009, 187.1987) -> (111.7024, 187.2506)
  line L2452 (111.7024, 187.2506) -> (111.9108, 187.2823)
  line L2453 (111.9108, 187.2823) -> (112.1255, 187.2931)
  line L2454 (112.1255, 187.2931) -> (112.3401, 187.2823)
  line L2455 (112.3401, 187.2823) -> (112.5489, 187.2506)
  line L2456 (112.5489, 187.2506) -> (112.7501, 187.1987)
  line L2457 (112.7501, 187.1987) -> (112.943, 187.1281)
  line L2458 (112.943, 187.1281) -> (113.1266, 187.0397)
  line L2459 (113.1266, 187.0397) -> (113.2995, 186.9345)
  line L2460 (113.2995, 186.9345) -> (113.4611, 186.8137)
  line L2461 (113.4611, 186.8137) -> (113.6103, 186.6782)
  line L2462 (113.6103, 186.6782) -> (113.746, 186.529)
  line L2463 (113.746, 186.529) -> (113.867, 186.3673)
  line L2464 (113.867, 186.3673) -> (113.972, 186.1941)
  line L2465 (113.972, 186.1941) -> (114.0606, 186.0107)
  line L2466 (114.0606, 186.0107) -> (114.1312, 185.8178)
  line L2467 (114.1312, 185.8178) -> (114.1829, 185.6164)
  line L2468 (114.1829, 185.6164) -> (114.2146, 185.408)
  line L2469 (114.2146, 185.408) -> (114.2256, 185.1932)
  line L2470 (114.2256, 185.1932) -> (114.2146, 184.9785)
  line L2471 (114.2146, 184.9785) -> (114.1829, 184.7699)
  line L2472 (114.1829, 184.7699) -> (114.1312, 184.5688)
  line L2473 (114.1312, 184.5688) -> (114.0606, 184.3758)
  line L2474 (114.0606, 184.3758) -> (113.972, 184.1922)
  line L2475 (113.972, 184.1922) -> (113.867, 184.0191)
  line L2476 (113.867, 184.0191) -> (113.746, 183.8573)
  line L2477 (113.746, 183.8573) -> (113.6103, 183.7083)
  line L2478 (113.6103, 183.7083) -> (113.4611, 183.5728)
  line L2479 (113.4611, 183.5728) -> (113.2995, 183.4519)
  line L2480 (113.2995, 183.4519) -> (113.1266, 183.3466)
  line L2481 (113.1266, 183.3466) -> (112.943, 183.2582)
  line L2482 (112.943, 183.2582) -> (112.7501, 183.1876)
  line L2483 (112.7501, 183.1876) -> (112.5489, 183.1359)
  line L2484 (112.5489, 183.1359) -> (112.3401, 183.1041)
  line L2485 (112.3401, 183.1041) -> (112.1255, 183.0932)
  line L2486 (112.1255, 183.0932) -> (111.9108, 183.1041)
  line L2487 (111.9108, 183.1041) -> (111.7024, 183.1359)
  line L2488 (111.7024, 183.1359) -> (111.5009, 183.1876)
  line L2489 (111.5009, 183.1876) -> (111.3079, 183.2582)
  line L2490 (111.3079, 183.2582) -> (111.1243, 183.3466)
  line L2491 (111.1243, 183.3466) -> (110.9514, 183.4519)
  line L2492 (110.9514, 183.4519) -> (110.7898, 183.5728)
  line L2493 (110.7898, 183.5728) -> (110.6406, 183.7083)
  line L2494 (110.6406, 183.7083) -> (110.5049, 183.8573)
  line L2495 (110.5049, 183.8573) -> (110.384, 184.0191)
  line L2496 (110.384, 184.0191) -> (110.2789, 184.1922)
  line L2497 (110.2789, 184.1922) -> (110.1903, 184.3758)
  line L2498 (110.1903, 184.3758) -> (110.1197, 184.5688)
  line L2499 (110.1197, 184.5688) -> (110.068, 184.7699)
  line L2500 (110.068, 184.7699) -> (110.0363, 184.9785)
  line L2501 (110.0363, 184.9785) -> (110.0253, 185.1932)
  line L2502 (40.0355, 185.1932) -> (40.0463, 185.408)
  line L2503 (40.0463, 185.408) -> (40.0782, 185.6164)
  line L2504 (40.0782, 185.6164) -> (40.1299, 185.8178)
  line L2505 (40.1299, 185.8178) -> (40.2005, 186.0107)
  line L2506 (40.2005, 186.0107) -> (40.289, 186.1941)
  line L2507 (40.289, 186.1941) -> (40.3941, 186.3673)
  line L2508 (40.3941, 186.3673) -> (40.515, 186.529)
  line L2509 (40.515, 186.529) -> (40.6506, 186.6782)
  line L2510 (40.6506, 186.6782) -> (40.7997, 186.8137)
  line L2511 (40.7997, 186.8137) -> (40.9613, 186.9345)
  line L2512 (40.9613, 186.9345) -> (41.1344, 187.0397)
  line L2513 (41.1344, 187.0397) -> (41.3181, 187.1281)
  line L2514 (41.3181, 187.1281) -> (41.511, 187.1987)
  line L2515 (41.511, 187.1987) -> (41.7122, 187.2506)
  line L2516 (41.7122, 187.2506) -> (41.9208, 187.2823)
  line L2517 (41.9208, 187.2823) -> (42.1354, 187.2931)
  line L2518 (42.1354, 187.2931) -> (42.3502, 187.2823)
  line L2519 (42.3502, 187.2823) -> (42.5586, 187.2506)
  line L2520 (42.5586, 187.2506) -> (42.76, 187.1987)
  line L2521 (42.76, 187.1987) -> (42.9529, 187.1281)
  line L2522 (42.9529, 187.1281) -> (43.1364, 187.0397)
  line L2523 (43.1364, 187.0397) -> (43.3097, 186.9345)
  line L2524 (43.3097, 186.9345) -> (43.4712, 186.8137)
  line L2525 (43.4712, 186.8137) -> (43.6204, 186.6782)
  line L2526 (43.6204, 186.6782) -> (43.756, 186.529)
  line L2527 (43.756, 186.529) -> (43.8769, 186.3673)
  line L2528 (43.8769, 186.3673) -> (43.982, 186.1941)
  line L2529 (43.982, 186.1941) -> (44.0705, 186.0107)
  line L2530 (44.0705, 186.0107) -> (44.1411, 185.8178)
  line L2531 (44.1411, 185.8178) -> (44.1928, 185.6164)
  line L2532 (44.1928, 185.6164) -> (44.2247, 185.408)
  line L2533 (44.2247, 185.408) -> (44.2355, 185.1932)
  line L2534 (44.2355, 185.1932) -> (44.2247, 184.9785)
  line L2535 (44.2247, 184.9785) -> (44.1928, 184.7699)
  line L2536 (44.1928, 184.7699) -> (44.1411, 184.5688)
  line L2537 (44.1411, 184.5688) -> (44.0705, 184.3758)
  line L2538 (44.0705, 184.3758) -> (43.982, 184.1922)
  line L2539 (43.982, 184.1922) -> (43.8769, 184.0191)
  line L2540 (43.8769, 184.0191) -> (43.756, 183.8573)
  line L2541 (43.756, 183.8573) -> (43.6204, 183.7083)
  line L2542 (43.6204, 183.7083) -> (43.4712, 183.5728)
  line L2543 (43.4712, 183.5728) -> (43.3097, 183.4519)
  line L2544 (43.3097, 183.4519) -> (43.1364, 183.3466)
  line L2545 (43.1364, 183.3466) -> (42.9529, 183.2582)
  line L2546 (42.9529, 183.2582) -> (42.76, 183.1876)
  line L2547 (42.76, 183.1876) -> (42.5586, 183.1359)
  line L2548 (42.5586, 183.1359) -> (42.3502, 183.1041)
  line L2549 (42.3502, 183.1041) -> (42.1354, 183.0932)
  line L2550 (42.1354, 183.0932) -> (41.9208, 183.1041)
  line L2551 (41.9208, 183.1041) -> (41.7122, 183.1359)
  line L2552 (41.7122, 183.1359) -> (41.511, 183.1876)
  line L2553 (41.511, 183.1876) -> (41.3181, 183.2582)
  line L2554 (41.3181, 183.2582) -> (41.1344, 183.3466)
  line L2555 (41.1344, 183.3466) -> (40.9613, 183.4519)
  line L2556 (40.9613, 183.4519) -> (40.7997, 183.5728)
  line L2557 (40.7997, 183.5728) -> (40.6506, 183.7083)
  line L2558 (40.6506, 183.7083) -> (40.515, 183.8573)
  line L2559 (40.515, 183.8573) -> (40.3941, 184.0191)
  line L2560 (40.3941, 184.0191) -> (40.289, 184.1922)
  line L2561 (40.289, 184.1922) -> (40.2005, 184.3758)
  line L2562 (40.2005, 184.3758) -> (40.1299, 184.5688)
  line L2563 (40.1299, 184.5688) -> (40.0782, 184.7699)
  line L2564 (40.0782, 184.7699) -> (40.0463, 184.9785)
  line L2565 (40.0463, 184.9785) -> (40.0355, 185.1932)
  line L2566 (26.0365, 185.1932) -> (26.0473, 185.408)
  line L2567 (26.0473, 185.408) -> (26.0792, 185.6164)
  line L2568 (26.0792, 185.6164) -> (26.1309, 185.8178)
  line L2569 (26.1309, 185.8178) -> (26.2015, 186.0107)
  line L2570 (26.2015, 186.0107) -> (26.2899, 186.1941)
  line L2571 (26.2899, 186.1941) -> (26.3951, 186.3673)
  line L2572 (26.3951, 186.3673) -> (26.516, 186.529)
  line L2573 (26.516, 186.529) -> (26.6516, 186.6782)
  line L2574 (26.6516, 186.6782) -> (26.8006, 186.8137)
  line L2575 (26.8006, 186.8137) -> (26.9624, 186.9345)
  line L2576 (26.9624, 186.9345) -> (27.1355, 187.0397)
  line L2577 (27.1355, 187.0397) -> (27.3191, 187.1281)
  line L2578 (27.3191, 187.1281) -> (27.512, 187.1987)
  line L2579 (27.512, 187.1987) -> (27.7132, 187.2506)
  line L2580 (27.7132, 187.2506) -> (27.9218, 187.2823)
  line L2581 (27.9218, 187.2823) -> (28.1364, 187.2931)
  line L2582 (28.1364, 187.2931) -> (28.3512, 187.2823)
  line L2583 (28.3512, 187.2823) -> (28.5597, 187.2506)
  line L2584 (28.5597, 187.2506) -> (28.7609, 187.1987)
  line L2585 (28.7609, 187.1987) -> (28.954, 187.1281)
  line L2586 (28.954, 187.1281) -> (29.1374, 187.0397)
  line L2587 (29.1374, 187.0397) -> (29.3105, 186.9345)
  line L2588 (29.3105, 186.9345) -> (29.4723, 186.8137)
  line L2589 (29.4723, 186.8137) -> (29.6214, 186.6782)
  line L2590 (29.6214, 186.6782) -> (29.7568, 186.529)
  line L2591 (29.7568, 186.529) -> (29.8778, 186.3673)
  line L2592 (29.8778, 186.3673) -> (29.983, 186.1941)
  line L2593 (29.983, 186.1941) -> (30.0714, 186.0107)
  line L2594 (30.0714, 186.0107) -> (30.142, 185.8178)
  line L2595 (30.142, 185.8178) -> (30.1939, 185.6164)
  line L2596 (30.1939, 185.6164) -> (30.2255, 185.408)
  line L2597 (30.2255, 185.408) -> (30.2364, 185.1932)
  line L2598 (30.2364, 185.1932) -> (30.2255, 184.9785)
  line L2599 (30.2255, 184.9785) -> (30.1939, 184.7699)
  line L2600 (30.1939, 184.7699) -> (30.142, 184.5688)
  line L2601 (30.142, 184.5688) -> (30.0714, 184.3758)
  line L2602 (30.0714, 184.3758) -> (29.983, 184.1922)
  line L2603 (29.983, 184.1922) -> (29.8778, 184.0191)
  line L2604 (29.8778, 184.0191) -> (29.7568, 183.8573)
  line L2605 (29.7568, 183.8573) -> (29.6214, 183.7083)
  line L2606 (29.6214, 183.7083) -> (29.4723, 183.5728)
  line L2607 (29.4723, 183.5728) -> (29.3105, 183.4519)
  line L2608 (29.3105, 183.4519) -> (29.1374, 183.3466)
  line L2609 (29.1374, 183.3466) -> (28.954, 183.2582)
  line L2610 (28.954, 183.2582) -> (28.7609, 183.1876)
  line L2611 (28.7609, 183.1876) -> (28.5597, 183.1359)
  line L2612 (28.5597, 183.1359) -> (28.3512, 183.1041)
  line L2613 (28.3512, 183.1041) -> (28.1364, 183.0932)
  line L2614 (28.1364, 183.0932) -> (27.9218, 183.1041)
  line L2615 (27.9218, 183.1041) -> (27.7132, 183.1359)
  line L2616 (27.7132, 183.1359) -> (27.512, 183.1876)
  line L2617 (27.512, 183.1876) -> (27.3191, 183.2582)
  line L2618 (27.3191, 183.2582) -> (27.1355, 183.3466)
  line L2619 (27.1355, 183.3466) -> (26.9624, 183.4519)
  line L2620 (26.9624, 183.4519) -> (26.8006, 183.5728)
  line L2621 (26.8006, 183.5728) -> (26.6516, 183.7083)
  line L2622 (26.6516, 183.7083) -> (26.516, 183.8573)
  line L2623 (26.516, 183.8573) -> (26.3951, 184.0191)
  line L2624 (26.3951, 184.0191) -> (26.2899, 184.1922)
  line L2625 (26.2899, 184.1922) -> (26.2015, 184.3758)
  line L2626 (26.2015, 184.3758) -> (26.1309, 184.5688)
  line L2627 (26.1309, 184.5688) -> (26.0792, 184.7699)
  line L2628 (26.0792, 184.7699) -> (26.0473, 184.9785)
  line L2629 (26.0473, 184.9785) -> (26.0365, 185.1932)
  line L2630 (12.0344, 185.1932) -> (12.0453, 185.408)